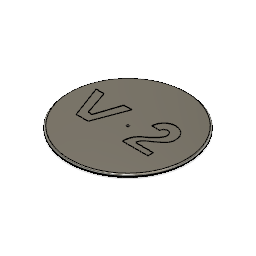
SkjotaraHjol2 v4 (Autodesk Fusion 360 design; units mm, degrees)
Autodesk Fusion 360 part; units mm, degrees
sketch "Sketch1" plane through (0, 0, 0) normal (0, 1, 0) x (1, 0, 0)
  circle A0 centre (0, 0) radius 150
  dimension "d1" = 300
  constraint coincident A0.centre origin
  measures "d1" diameter of A0
extrude "Extrude1" add sketch "Sketch1" along normal blind 10
fillet "Fillet1" radius 4 1 edges at (-139.8491, 10, 54.2423)
fillet "Fillet2" radius 4 1 edges at (-139.8491, 0, 54.2423)
sketch "Sketch2" plane through (0, 0, 0) normal (0, -1, 0) x (1, 0, 0)
  circle A0 centre (0, 0) radius 146
sketch "Sketch3" plane through (0, 0, 0) normal (0, 1, 0) x (1, 0, 0)
  circle A0 centre (0, 0) radius 1.555
  dimension "d12" = 3.11
  constraint coincident A0.centre origin
  measures "d12" diameter of A0
extrude "Extrude2" cut sketch "Sketch3" along normal blind 11
sketch "Sketch4" plane through (0, 10, 0) normal (0, 1, 0) x (-1, 0, 0)
  circle A0 centre (0, 0) radius 1.555
  circle A1 centre (0, 0) radius 146
  line L0 (120, -40) -> (90, 40)
  line L1 (90, 40) -> (60, 40)
  line L2 (60, 40) -> (30, -40)
  line L3 (30, -40) -> (50, -40)
  line L4 (50, -40) -> (70, 20)
  line L5 (70, 20) -> (80, 20)
  line L6 (80, 20) -> (100, -40)
  line L7 (100, -40) -> (120, -40)
  line L8 (-30, -30) -> (-50, -30)
  arc A2 (-70, -30) -> (-50, -30) centre (-60, -30) ccw
  arc A3 (-90, -30) -> (-30, -30) centre (-60, -30) ccw
  spline S0 degree 5 poles (-70, -30) (-70.0634, -29.7236) (-70.1723, -29.1665) (-70.2819, -28.3178) (-70.3207, -27.1599) (-70.1889, -25.6686) (-69.8751, -24.1335) (-69.376, -22.5546) (-68.6884, -20.9329) (-67.8134, -19.2713) (-66.7594, -17.5764) (-65.547, -15.8596) (-64.2094, -14.1377) (-62.7845, -12.4293) (-61.3071, -10.7508) (-59.8021, -9.1139) (-58.2756, -7.5214) (-56.7101, -5.965) (-55.0757, -4.4303) (-53.3406, -2.9009) (-51.4819, -1.3633) (-49.4955, 0.189) (-47.4087, 1.7499) (-45.2741, 3.3045) (-43.1564, 4.8358) (-41.1228, 6.3305) (-39.2311, 7.7847) (-37.5194, 9.21) (-35.9935, 10.6403) (-34.6345, 12.1238) (-33.4107, 13.7116) (-32.2874, 15.4473) (-31.2375, 17.3568) (-30.2526, 19.4371) (-29.3384, 21.6635) (-28.5106, 23.9969) (-27.7898, 26.3921) (-27.1977, 28.8042) (-26.7512, 31.1975) (-26.4611, 33.5493) (-26.3334, 35.8458) (-26.3632, 37.6333) (-26.46, 38.9452) (-26.5577, 39.8069) (-26.6147, 40.2346) knots 0 0 0 0 0 0 0.025 0.05 0.075 0.1 0.125 0.15 0.175 0.2 0.225 0.25 0.275 0.3 0.325 0.35 0.375 0.4 0.425 0.45 0.475 0.5 0.525 0.55 0.575 0.6 0.625 0.65 0.675 0.7 0.725 0.75 0.775 0.8 0.825 0.85 0.875 0.9 0.925 0.95 0.975 1 1 1 1 1 1
  spline S1 degree 5 poles (-90, -30) (-90.0442, -29.7838) (-90.1209, -29.3378) (-90.2007, -28.6279) (-90.2365, -27.5994) (-90.1634, -26.1809) (-89.9721, -24.6411) (-89.6627, -23.0046) (-89.2357, -21.3104) (-88.6909, -19.6034) (-88.0272, -17.9257) (-87.2416, -16.31) (-86.328, -14.7695) (-85.2785, -13.2964) (-84.0856, -11.8706) (-82.7446, -10.4656) (-81.2559, -9.0553) (-79.6283, -7.6214) (-77.8793, -6.1572) (-76.0322, -4.6645) (-74.114, -3.1522) (-72.1524, -1.6337) (-70.1735, -0.1252) (-68.1991, 1.3564) (-66.2443, 2.796) (-64.3188, 4.1811) (-62.4289, 5.504) (-60.5798, 6.763) (-58.7772, 7.9643) (-57.0291, 9.1229) (-55.3486, 10.266) (-53.7526, 11.4282) (-52.2604, 12.6449) (-50.8915, 13.9443) (-49.6636, 15.3415) (-48.5909, 16.8301) (-47.6823, 18.3787) (-46.9432, 19.942) (-46.3762, 21.4701) (-45.982, 22.9167) (-45.7603, 24.2509) (-45.7206, 25.2167) (-45.768, 25.8818) (-45.8338, 26.299) (-45.8753, 26.5009) knots 0 0 0 0 0 0 0.025 0.05 0.075 0.1 0.125 0.15 0.175 0.2 0.225 0.25 0.275 0.3 0.325 0.35 0.375 0.4 0.425 0.45 0.475 0.5 0.525 0.55 0.575 0.6 0.625 0.65 0.675 0.7 0.725 0.75 0.775 0.8 0.825 0.85 0.875 0.9 0.925 0.95 0.975 1 1 1 1 1 1
  line L9 (-45.8753, 26.5009) -> (-90, 26.5009)
  line L10 (-90, 26.5009) -> (-90, 40)
  line L11 (-90, 40) -> (-26.6147, 40.2346)
  point P0 (-70, -24.8518)
  point P1 (-67, -18)
  point P2 (-60, -9.3422)
  point P3 (-51, -1)
  point P4 (-39, 8)
  point P5 (-32.2588, 15.5698)
  point P6 (-27.4521, 27.8408)
  point P7 (-90, -25)
  point P8 (-87.5787, -17.0448)
  point P9 (-81.7168, -9.508)
  point P10 (-70, 0)
  point P11 (-58.1016, 8.4127)
  point P12 (-50, 15)
  point P13 (-46.2103, 22.1464)
  constraint horizontal L1
  constraint parallel L1 L3
  constraint parallel L3 L5
  constraint parallel L5 L7
  constraint horizontal L8
  constraint coincident A2.centre A3.centre
  constraint horizontal L9
  constraint perpendicular L9 L10
extrude "Extrude3" cut sketch "Sketch4" against normal blind 1 contours L0 L1 L2 L3 L4 L5 L6 L7 | L8 A2 A3 S0 S1 L9 L10 L11
scale "Scale1" factor 0.5 about (-120, 10, -40) bodies 1
sketch "Sketch5" plane through (0, 10, 0) normal (0, 1, 0) x (-1, 0, 0)
  line L0 (105, 0) -> (120, -40)
  line L1 (120, -40) -> (110, -40)
  line L2 (110, -40) -> (100, -10)
  line L3 (100, -10) -> (95, -10)
  line L4 (95, -10) -> (85, -40)
  line L5 (85, -40) -> (75, -40)
  line L6 (75, -40) -> (90, 0)
  line L7 (90, 0) -> (105, 0)
  line L8 (35, -35) -> (45, -35)
  arc A0 (15, -35) -> (45, -35) centre (30, -35) ccw
  spline S0 degree 5 poles (15, -35) (14.9779, -34.8919) (14.9396, -34.6689) (14.8997, -34.3139) (14.8818, -33.7997) (14.9183, -33.0904) (15.0139, -32.3206) (15.1686, -31.5023) (15.3821, -30.6552) (15.6545, -29.8017) (15.9864, -28.9629) (16.3792, -28.155) (16.836, -27.3848) (17.3607, -26.6482) (17.9572, -25.9353) (18.6277, -25.2328) (19.372, -24.5277) (20.1858, -23.8107) (21.0604, -23.0786) (21.9839, -22.3322) (22.943, -21.5761) (23.9238, -20.8169) (24.9133, -20.0626) (25.9004, -19.3218) (26.8778, -18.602) (27.8406, -17.9094) (28.7856, -17.248) (29.7101, -16.6185) (30.6114, -16.0179) (31.4854, -15.4385) (32.3257, -14.867) (33.1237, -14.2859) (33.8698, -13.6776) (34.5542, -13.0279) (35.1682, -12.3293) (35.7046, -11.585) (36.1589, -10.8107) (36.5284, -10.029) (36.8119, -9.265) (37.009, -8.5416) (37.1199, -7.8746) (37.1397, -7.3916) (37.116, -7.0591) (37.0831, -6.8505) (37.0623, -6.7495) knots 0 0 0 0 0 0 0.025 0.05 0.075 0.1 0.125 0.15 0.175 0.2 0.225 0.25 0.275 0.3 0.325 0.35 0.375 0.4 0.425 0.45 0.475 0.5 0.525 0.55 0.575 0.6 0.625 0.65 0.675 0.7 0.725 0.75 0.775 0.8 0.825 0.85 0.875 0.9 0.925 0.95 0.975 1 1 1 1 1 1
  line L9 (37.0623, -6.7495) -> (15, -6.7495)
  line L10 (15, -6.7495) -> (15, 0)
  line L11 (15, 0) -> (46.6926, 0.1173)
  spline S1 degree 5 poles (46.6926, 0.1173) (46.7212, -0.0965) (46.77, -0.5274) (46.8184, -1.1833) (46.8333, -2.0771) (46.7694, -3.2253) (46.6244, -4.4012) (46.4012, -5.5979) (46.1051, -6.804) (45.7447, -8.0015) (45.3308, -9.1683) (44.8737, -10.2814) (44.3812, -11.3216) (43.8563, -12.2763) (43.2946, -13.1442) (42.6827, -13.9381) (42.0033, -14.6798) (41.2403, -15.395) (40.3845, -16.1076) (39.4386, -16.8347) (38.4218, -17.5821) (37.363, -18.3478) (36.2956, -19.1251) (35.2523, -19.9055) (34.259, -20.6816) (33.3297, -21.4504) (32.4621, -22.2152) (31.645, -22.9825) (30.8622, -23.7607) (30.099, -24.5569) (29.3464, -25.3754) (28.6078, -26.2146) (27.8953, -27.0689) (27.2265, -27.9298) (26.6203, -28.7882) (26.0933, -29.6357) (25.6558, -30.4664) (25.312, -31.2773) (25.0624, -32.0667) (24.9055, -32.8343) (24.8397, -33.5799) (24.859, -34.1589) (24.9139, -34.5833) (24.9683, -34.8618) (25, -35) knots -1 -1 -1 -1 -1 -1 -0.975 -0.95 -0.925 -0.9 -0.875 -0.85 -0.825 -0.8 -0.775 -0.75 -0.725 -0.7 -0.675 -0.65 -0.625 -0.6 -0.575 -0.55 -0.525 -0.5 -0.475 -0.45 -0.425 -0.4 -0.375 -0.35 -0.325 -0.3 -0.275 -0.25 -0.225 -0.2 -0.175 -0.15 -0.125 -0.1 -0.075 -0.05 -0.025 0 0 0 0 0 0
  arc A1 (25, -35) -> (35, -35) centre (30, -35) ccw
  circle A2 centre (60, -20) radius 0.7775
  circle A3 centre (60, -20) radius 73
  circle A4 centre (60, -20) radius 1.555
  dimension "d18" = 3.11
  constraint concentric A2 A4
  measures "d18" diameter of A4
extrude "Extrude4" cut sketch "Sketch5" against normal blind 11 contours A4
